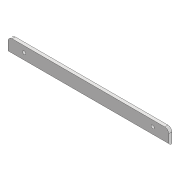
# Autodesk Inventor part: SlipersLåda 211018009
Saved by Autodesk Inventor 2020 (Build 240168000, 168)
## iProperties
Created: 2021-10-19
Part Number: SlipersLåda 211018009
Material: Generic
Document SubType Name: Modeling
Designer: dicpet001
Density: 1 g/cm^3
Appearance: Default
Author: dicpet001
Autodesk Inventor part; units mm, degrees
ref_plane "YZ Plane" through (0, 0, 0) normal (1, 0, 0) x (0, 1, 0)
ref_plane "XZ Plane" through (0, 0, 0) normal (0, 1, 0) x (-1, 0, 0)
ref_plane "XY Plane" through (0, 0, 0) normal (0, 0, 1) x (1, 0, 0)
sketch "Sketch1" plane through (0, 0, 0) normal (0, 0, 1) x (1, 0, 0)
  line L0 (0, 26.9853) -> (0, -24.9142) projected
  line L1 (-282.8995, 0) -> (282.8995, 0) projected
  line L2 (-190, 17.5) -> (190, 17.5)
  line L3 (200, 7.5) -> (200, -17.5)
  line L4 (200, -17.5) -> (-200, -17.5)
  line L5 (-200, -17.5) -> (-200, 7.5)
  arc A0 (-190, 17.5) -> (-200, 7.5) centre (-190, 7.5) ccw
  arc A1 (200, 7.5) -> (190, 17.5) centre (190, 7.5) ccw
  circle A2 centre (-160, 2.5) radius 4
  circle A3 centre (160, 2.5) radius 4
  point P0 (0, 0)
  point P1 (-200, 17.5)
  point P2 (200, 17.5)
  dimension "d0" = 35
  dimension "d1" = 400
  dimension "d2" = 10
  dimension "d3" = 8
  dimension "d4" = 160
  dimension "d5" = 20
  constraints: 8 end point, 4 centre point, 4 point on circle, 4 point on line, 4 tangent, 2 equal radius, 2 parallel, 1 horizontal, 1 perpendicular, 1 symmetric about line, 2 other
  measures "d0" distance of L4.end point (-200, 17.5)
  measures "d1" distance of point (-200, 17.5) point (200, 17.5)
  measures "d2" radius of A0
  measures "d3" diameter of A2
  measures "d4" distance from line of L0 A2.centre
  measures "d5" distance from line of L4 A2.centre
extrude "Extrusion1" add sketch "Sketch1" against normal blind 8 contours L2 A1 L3 L1 A3 L0 | L0 L1 A2 L5 A0 L2 | L1 A3 L3 L4 L0 | L0 L4 L5 L1 A2
chamfer "Chamfer1" distance 4 angle 45 1 edges at (0, -17.5, 0)
body "Solid1"
